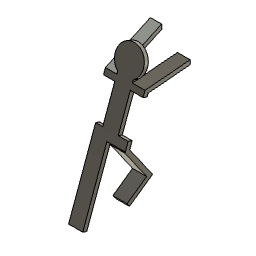
Plant Pusher v1 (Autodesk Fusion 360 design; units mm, degrees)
Autodesk Fusion 360 part; units mm, degrees
sketch "Sketch1" plane through (0, 0, 0) normal (0, 1, 0) x (1, 0, 0)
  line L0 (0, 0) -> (10, 0)
  line L1 (10, 0, 0) -> (10, -46.9846, 17.101)
  line L2 (10, -46.9846, 17.101) -> (0, -46.9846, 17.101)
  line L3 (0, -46.9846, 17.101) -> (0, 0, 0)
  dimension "d1" = 10
  dimension "d2" = 50
  constraint coincident L0.start origin
  measures "d1" distance of L0.start L0.end
extrude "Extrude1" add sketch "Sketch1" along normal blind 3 contours L0 L1 L2 L3 in plane through (0, 0, 0) normal (0, 0.939693, -0.34202) makes body 1
sketch "Sketch2" plane through (0, 0, 0) normal (0, -0.939693, 0.34202) x (1, 0, 0)
  line L0 (10, 50) -> (0, 50)
  line L1 (0, 50) -> (0, 0)
  line L2 (0, 0) -> (10, 0)
  line L3 (10, 0) -> (10, 50)
  line L4 (13, 50) -> (13, 47)
  line L5 (10, 47) -> (10, 50)
  line L6 (13, 50) -> (23, 50)
  line L7 (23, 50) -> (23, 20)
  line L8 (23, 20) -> (13, 20)
  line L9 (13, 20) -> (13, 50)
  dimension "d5" = 3
  dimension "d6" = 3
  dimension "d7" = 10
  constraint vertical L4
  constraint vertical L5
  constraint coincident L0.start L3.end
  constraint horizontal L6
  constraint vertical L7
  constraint horizontal L8
  constraint vertical L9
  measures "d5" distance of L0.start L4.start
  measures "d6" distance of L0.start L5.start
  measures "d7" distance of L4.start L6.end
extrude "Extrude2" add sketch "Sketch2" against normal blind 3 separate body contours L4 L6 L7 L8 L9 makes body 2
move_body "Move1" bodies 2 to x (1, 0, 0) y (0, 0.573576, 0.819152) z (0, -0.819152, 0.573576) at (0, 45.4412, 5.6533)
sketch "Sketch3" plane through (0, 0.822, -1.1739) normal (0, 0.573576, -0.819152) x (-1, 0, 0)
  line L0 (-23, 40.4658) -> (-13, 40.4658)
  line L1 (-13, 40.4658) -> (-13, 43.4658)
  line L2 (-13, 43.4658) -> (-23, 43.4658)
  line L3 (-23, 43.4658) -> (-23, 40.4658)
  line L4 (-23, 43.4658) -> (-13, 43.4658)
  line L5 (-13, 43.4658) -> (-13, 23.4658)
  line L6 (-13, 23.4658) -> (-23, 23.4658)
  line L7 (-23, 23.4658) -> (-23, 43.4658)
  dimension "d11" = 20
  constraint horizontal L4
  constraint vertical L5
  constraint horizontal L6
  constraint vertical L7
  constraint coincident L2.end L3.start
  measures "d11" distance of L2.end L6.end
extrude "Extrude3" add sketch "Sketch3" against normal blind 3 contours L0 L5 L6 L7 bodies 2
sketch "Sketch4" plane through (0, 17.101, 46.9846) normal (0, 0.34202, 0.939693) x (-1, 0, 0)
  line L0 (0, 0) -> (-10, 0)
  line L1 (-10, 0) -> (-10, -3)
  line L2 (-10, -3) -> (0, -3)
  line L3 (0, -3) -> (0, 0)
  line L4 (0, -3) -> (-23, -3)
  line L5 (-23, -3) -> (-23, 0)
  line L6 (-23, 0) -> (0, 0)
  line L7 (0, 0) -> (0, -3)
  constraint horizontal L4
  constraint vertical L5
  constraint horizontal L6
  constraint vertical L7
  constraint coincident L2.end L3.start
extrude "Extrude4" add sketch "Sketch4" along normal blind 6 bodies 1 2
sketch "Sketch5" plane through (0, 0, 0) normal (0, -0.939693, 0.34202) x (1, 0, 0)
  line L0 (0, 56) -> (0, 0)
  line L1 (0, 0) -> (10, 0)
  line L2 (10, 0) -> (10, 50)
  line L3 (10, 50) -> (23, 50)
  line L4 (23, 50) -> (23, 56)
  line L5 (23, 56) -> (0, 56)
  line L6 (5, 56) -> (16, 56)
  line L7 (16, 56) -> (16, 88)
  line L8 (16, 88) -> (5, 88)
  line L9 (5, 88) -> (5, 56)
  dimension "d16" = 11
  dimension "d17" = 32
  constraint horizontal L6
  constraint vertical L7
  constraint horizontal L8
  constraint vertical L9
  constraint coincident L5 L6.start
  measures "d16" distance of L6.start L6.end
  measures "d17" distance of L6.start L8.end
extrude "Extrude5" add sketch "Sketch5" against normal blind 3 contours L5 L6 L7 L8 L9 bodies 1
sketch "Sketch6" plane through (0, 0, 0) normal (0, -0.939693, 0.34202) x (1, 0, 0)
  line L0 (0, 56) -> (0, 0)
  line L1 (0, 0) -> (10, 0)
  line L2 (10, 0) -> (10, 50)
  line L3 (10, 50) -> (23, 50)
  line L4 (23, 50) -> (23, 56)
  line L5 (23, 56) -> (16, 56)
  line L6 (16, 56) -> (16, 88)
  line L7 (16, 88) -> (5, 88)
  line L8 (5, 88) -> (5, 56)
  line L9 (5, 56) -> (0, 56)
  circle A0 centre (10.5, 95.042) radius 10
  dimension "d20" = 20
  measures "d20" diameter of A0
extrude "Extrude6" add sketch "Sketch6" against normal blind 3 contours L6 L7 L8 A0 picked at (10.3277, 93.6762) bodies 1
sketch "Sketch7" plane through (0, 0, 0) normal (0, -0.939693, 0.34202) x (1, 0, 0)
  line L0 (0, 56) -> (0, 0)
  line L1 (0, 0) -> (10, 0)
  line L2 (10, 0) -> (10, 50)
  line L3 (10, 50) -> (23, 50)
  line L4 (23, 50) -> (23, 56)
  line L5 (23, 56) -> (16, 56)
  line L6 (16, 56) -> (16, 86.6903)
  arc A0 (16, 86.6903) -> (5, 86.6903) centre (10.5, 95.042) ccw
  line L7 (5, 86.6903) -> (5, 56)
  line L8 (5, 56) -> (0, 56)
  line L9 (-3, 85) -> (25, 85)
  line L10 (25, 85) -> (25, 81)
  line L11 (25, 81) -> (-3, 81)
  line L12 (-3, 81) -> (-3, 85)
  constraint horizontal L9
  constraint vertical L10
  constraint horizontal L11
  constraint vertical L12
extrude "Extrude7" add sketch "Sketch7" against normal blind 3 contours L7 L9 L11 L12 | L6 L7 L9 L11 | L6 L9 L10 L11 bodies 1
sketch "Sketch8" plane through (0, 29.0717, 79.8739) normal (0, 0.34202, 0.939693) x (-1, 0, 0)
  line L0 (-5, 0) -> (-5, -3)
  line L1 (-5, -3) -> (3, -3)
  line L2 (3, -3) -> (3, 0)
  line L3 (3, 0) -> (-5, 0)
  line L4 (-5, 0) -> (3, 0)
  line L5 (3, 0, 0) -> (3, -24.7487, 24.7487)
  line L6 (3, -24.7487, 24.7487) -> (-5, -24.7487, 24.7487)
  line L7 (-5, -24.7487, 24.7487) -> (-5, 0, 0)
  dimension "d25" = 35
  constraint coincident L0.start L3.end
sketch "Sketch9" plane through (1, 44.9321, 87.2697) normal (0, -0.422618, 0.906308) x (1, 0, 0)
sketch "Sketch10" plane through (0, 0, 0) normal (1, 0, 0) x (0, 1, 0)
  line L0 (41, 0) -> (100, 0)
  line L1 (100, 0) -> (100, 100)
  line L2 (100, 100) -> (41, 100)
  line L3 (41, 100) -> (41, 0)
  constraint horizontal L0
  constraint vertical L1
  constraint horizontal L2
  constraint vertical L3
extrude "Extrude8" add sketch "Sketch10" along normal blind 50 separate body makes body 3
move_body "Move2" bodies 3 to x (1, 0, 0) y (0, 1, 0) z (0, 0, 1) at (0, 30, 0)
extrude "Extrude9" add sketch "Sketch8" against normal blind 3 contours L3 L4 L5 L6 L7 in plane through (0, 29.0717, 79.8739) normal (0, -0.422618, 0.906308) bodies 1
sketch "Sketch11" plane through (0, 29.0717, 79.8739) normal (0, 0.34202, 0.939693) x (-1, 0, 0)
  line L0 (-16, -3) -> (-16, 0)
  line L1 (-16, 0) -> (-25, 0)
  line L2 (-25, 0) -> (-25, -3)
  line L3 (-25, -3) -> (-16, -3)
  line L4 (-16, 0) -> (-25, 0)
  line L5 (-25, 0, 0) -> (-25, -36.2523, 16.9047)
  line L6 (-25, -36.2523, 16.9047) -> (-16, -36.2523, 16.9047)
  line L7 (-16, -36.2523, 16.9047) -> (-16, 0, 0)
  dimension "d30" = 40
  constraint coincident L0.end L1.start
extrude "Extrude10" add sketch "Sketch11" against normal blind 3 contours L1 L4 L5 L6 L7 in plane through (0, 29.0717, 79.8739) normal (0, -0.087156, 0.996195) bodies 1
move_face "MoveFace1" by (0, 20, 0) 4 faces at (50, 90.6667, 66.6667) (16.6667, 71, 66.6667) (16.6667, 110.3333, 100) (0, 90.6667, 66.6667) on bodies 3
extrude "Extrude11" cut 1 faces at (16.6667, 91, 66.6667) along direction (0, -1, 0) blind 30 on bodies 3 bodies 1
delete_face "DeleteFace1" 6 faces at (50, 104, 66.6667) (16.6667, 91, 66.6667) (33.3333, 117, 100) (0, 104, 66.6667) (33.3333, 130, 66.6667) (33.3333, 104, 0) on bodies 3
